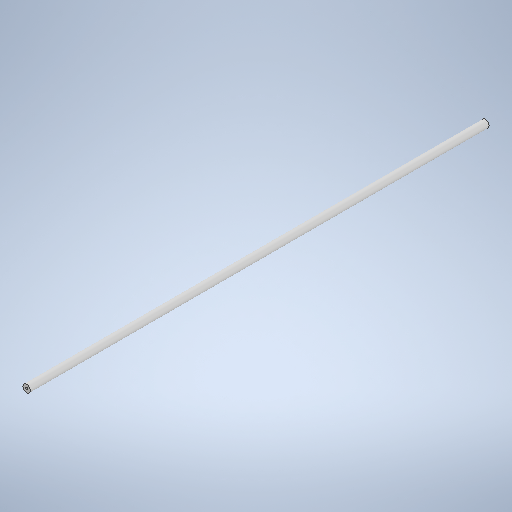
# Autodesk Inventor part: walek_liniowy_fi16_L1000
Saved by Autodesk Inventor 2025.2 (Build 292293000, 293)
## iProperties
Created: 2025-03-20
Part Number: walek_liniowy_fi16_L1000
Material: Ogólny
Document SubType Name: Modeling
Designer: rango
Density: 1 g/cm^3
Appearance: Domyślna
Author: rango
Autodesk Inventor part; units mm, degrees
ref_plane "YZ Plane" through (0, 0, 0) normal (1, 0, 0) x (0, 1, 0)
ref_plane "XZ Plane" through (0, 0, 0) normal (0, 1, 0) x (-1, 0, 0)
ref_plane "XY Plane" through (0, 0, 0) normal (0, 0, 1) x (1, 0, 0)
sketch "Szkic1" plane through (0, 0, 0) normal (0, 0, 1) x (1, 0, 0)
  circle A0 centre (0, 0) radius 8
  line L0 (0, 8) -> (0, 0) construction
  dimension "d0" = 16
  constraints: 2 end point, 1 coincident, 1 vertical, 1 vertical alignment, 2 other
extrude "Wyciągnięcie proste1" add sketch "Szkic1" along normal blind 1000
sketch "Szkic2" plane through (0, 0, 1000) normal (0, 0, 1) x (1, 0, 0)
  circle A0 centre (0, 0) radius 8 projected
  line L0 (0, 8) -> (0, -8)
  line L1 (-8, 0) -> (8, 0)
  constraints: 4 end point, 4 point on circle, 1 perpendicular, 1 vertical
hole "Otwór1" at (0, 0, 1000) direction (0, 0, -1) diameter 4.9784 depth 32 tip angle 118 thread size "1/4-20 UNC" class "2B" standard "ANSI Unified Screw Threads"
sketch "Szkic3" plane through (0, 0, 0) normal (0, 0, -1) x (-1, 0, 0)
  circle A0 centre (0, 0) radius 8 projected
  line L0 (0, 8) -> (0, -8)
  line L1 (-8, 0) -> (8, 0)
  constraints: 4 end point, 4 point on circle, 1 perpendicular, 1 vertical
hole "Otwór2" at (0, 0, 0) direction (0, 0, 1) diameter 4.9784 depth 32 tip angle 118 thread size "1/4-20 UNC" class "2B" standard "ANSI Unified Screw Threads"
